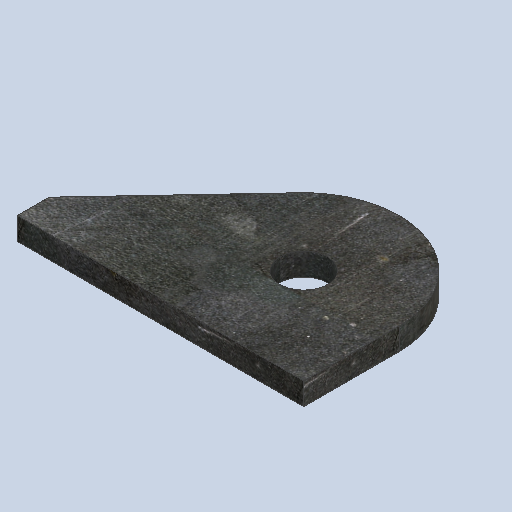
# Autodesk Inventor part: CSM-EB-EPP-001-PL-001
Saved by Autodesk Inventor 2023 (Build 270158000, 158)
## iProperties
RuleStatus: InUse
Created: 2023-05-12
Part Number: CSM-EB-EPP-001-PL-001
Material: Acero ASTM A36
Description: =PL <anchodesarrollo> x <largodesarrollo>, THK: <Grosor>
Document SubType Name: Sheet Metal
Designer: NELSON ORTIZ
Density: 7.85 g/cm^3
Sheet Metal Rule: Por defecto_mm
Appearance: Placa
Mass: 3067.93 g
Surface Area: 705.752 cm^2
Volume: 390.819 cm^3
Sheet Metal Width: 120,000 mm
Sheet Metal Length: 180,000 mm
Sheet Metal Area: 21600,000 mm^2
Flat Pattern Width: 12 cm
Flat Pattern Length: 18 cm
Flat Pattern Area: 216 cm^2
AfterDocOpen0: OPEN
areadesarrollo: 21600 mm^2
anchodesarrollo: 120 mm
largodesarrollo: 180 mm
Grosor: 9/16"
L: 180,000 mm
h_: 60,000 mm
epl: 14,000 mm
r: 60,000 mm
hole: 30,000 mm
hole_gr: 25,400 mm
a: 7,000 mm
b: 20,000 mm
eb: 7,000 mm
ton: 6,000 su
peso: 1,600 kg
grillete: 0,034 in
iTrigger0: 1,000 su
Author: NELSON ORTIZ
Keywords: 15
Comments: 4
Autodesk Inventor part; units mm, degrees
note: some values were not read from the file. Left out: dimensions or parameters whose unit could not be read.
ref_plane "YZ Plane" through (0, 0, 0) normal (1, 0, 0) x (0, 1, 0)
ref_plane "XZ Plane" through (0, 0, 0) normal (0, 1, 0) x (-1, 0, 0)
ref_plane "XY Plane" through (0, 0, 0) normal (0, 0, 1) x (1, 0, 0)
sketch "Boceto2" plane through (0, 0, 0) normal (0, 1, 0) x (-1, 0, 0)
  circle A0 centre (0, 0) radius 15
  arc A1 (-60, 0) -> (43.7033, -41.1099) centre (0, 0) ccw
  line L0 (43.7033, -41.1099) -> (120, 40)
  line L1 (120, 40) -> (120, 60)
  line L2 (120, 60) -> (-60, 60)
  line L3 (-60, 60) -> (-60, 0)
  line L4 (0, 0) -> (43.7033, -41.1099) construction
  line L5 (0, 0) -> (-60, 0) construction
  dimension "d7" = 60
  dimension "d8" = 20
  dimension "d9" = 60
  dimension "d10" = 180
  dimension "d11" = 30
  measures "d7" distance of L2.end L3.end
  measures "d8" distance of L0.end L1.end
  measures "d9" distance from line of L3 point (0, 0)
  measures "d10" distance of L1.end L2.end
  measures "d11" diameter of A0
extrude "Placa2" add sketch "Boceto2" along normal mid plane 14
equation "\"d7\" = h_"
equation "\"d8\" = b"
equation "\"d9\" = r"
equation "\"d10\" = L"
equation "\"d11\" = hole"
equation "\"d12\" = Grosor"
equation "\"Grosor\" = epl"
equation "\"Radio_pliegue\" = Grosor"
equation "\"Anchura_desahogo_plegado\" = Grosor"
equation "\"Profundidad_desahogo_plegado\" = 0.5 * Grosor"
equation "\"Tamaño_destalonado\" = 4 * Grosor"
equation "\"Remanente_mínimo\" = 2 * Grosor"
equation "\"Radiodetransición\" = Radio_pliegue"
equation "\"Tamaño_de_radio_de_Jacobi\" = Radio_pliegue"
equation "\"TamañoSeparación\" = Grosor"
equation "\"L\" = 180"
equation "\"epl\" = 14"
equation "\"h_\" = 60"
equation "\"r\" = 60"
equation "\"hole\" = 30"
equation "\"hole_gr\" = 25.4"
equation "\"a\" = 7"
equation "\"b\" = 20"
equation "\"eb\" = 7"
equation "\"grillete\" = 0.875"
